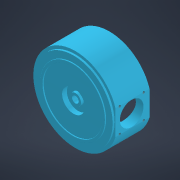
# Autodesk Inventor part: 008
Saved by Autodesk Inventor 2022 (Build 260153000, 153)
## iProperties
Created: 2021-11-17
Part Number: 008
Material: Steel, Carbon
Document SubType Name: Modeling
Designer: vinicius.miguel
Density: 7.85 g/cm^3
Appearance: Turquoise
Mass: 775.835 g
Surface Area: 314.081 cm^2
Volume: 98.8324 cm^3
Author: vinicius.miguel
Autodesk Inventor part; units mm, degrees
ref_plane "XZ Plane" through (0, 0, 0) normal (0, 1, 0) x (-1, 0, 0)
ref_plane "XY Plane" through (0, 0, 0) normal (0, 0, 1) x (1, 0, 0)
sketch "Sketch1" plane through (0, 0, 0) normal (0, 1, 0) x (-1, 0, 0)
  line L0 (0, 0) -> (0, 38)
  line L1 (-3.5, 30) -> (-15, 30)
  line L2 (-15, 30) -> (-15, 35)
  line L3 (-15, 35) -> (-34.45, 35)
  line L4 (-34.45, 35) -> (-34.45, 0)
  line L5 (-34.45, 0) -> (-44.45, 0)
  line L6 (-44.45, 0) -> (-44.45, 38)
  line L7 (-44.45, 38) -> (-34.5, 38)
  line L8 (-34.5, 38) -> (-34.5, 39)
  line L9 (-34.5, 39) -> (-31.5, 39)
  line L10 (-31.5, 39) -> (-31.5, 38)
  line L11 (-31.5, 38) -> (-12, 38)
  line L12 (-12, 33) -> (-3.5, 33)
  line L13 (-12, 38) -> (-12, 33)
  line L14 (-3.5, 33) -> (-3.5, 30)
  line L15 (-3.5, 33) -> (-3.5, 36)
  line L16 (-3.5, 36) -> (-6, 36)
  line L17 (-6, 36) -> (-6, 33)
  dimension "d5" = 69
  dimension "d6" = 3
  dimension "d7" = 1
  dimension "d8" = 88.9
  dimension "d10" = 3
  dimension "d11" = 5
  dimension "d12" = 30
  dimension "d37" = 10
  dimension "d64" = 38
  dimension "d74" = 7
  dimension "d75" = 24
  dimension "d76" = 3
  dimension "d77" = 2.5
  dimension "d78" = 3
  constraints: 36 end point, 16 perpendicular, 4 vertical, 2 horizontal alignment, 2 point on line
  measures "d5" diameter of L8 L0
  measures "d6" distance of L8.end L9.end
  measures "d7" distance of L9.end L10.end
  measures "d8" diameter of L6 L0
  measures "d10" distance between parallel lines of L11 L3
  measures "d11" distance of L1.end L2.end
  measures "d12" diameter of L2 L0
  measures "d37" distance between parallel lines of L6 L4
  measures "d64" distance of L5.end L6.end
  measures "d74" diameter of L14 L0
  measures "d75" diameter of L13 L0
  measures "d76" distance of L12.end L1.start
  measures "d77" distance of L15.end L16.end
  measures "d78" distance of L16.end L17.end
revolve "Revolution1" add sketch "Sketch1" angle 360 about axis through (0, 0, 0) along (0, 0, 1)
ref_plane "Work Plane1" through (44.45, 0, 19) normal (1, 0, 0) x (0, 1, 0)
sketch "Sketch7" plane through (44.45, 0, 19) normal (1, 0, 0) x (0, 1, 0)
  line L0 (34.45, 16) -> (-34.45, 16) projected
  line L1 (34.45, -19) -> (-34.45, -19) projected
  line L2 (34.45, 16) -> (-34.45, 16) projected
  line L3 (0, 16) -> (0, -19) construction
  line L4 (57.5, 28.575) -> (-57.5, 28.575)
  line L5 (-57.5, 28.575) -> (-57.5, -31.575)
  line L6 (-57.5, -31.575) -> (57.5, -31.575)
  line L7 (57.5, -31.575) -> (57.5, 28.575)
  line L8 (57.5, 28.575) -> (-57.5, -31.575) construction
  line L9 (-57.5, 28.575) -> (57.5, -31.575) construction
  point P0 (0, -1.5)
  dimension "d79" = 115
  dimension "d80" = 60.1501
  constraints: 14 end point, 4 midpoint, 2 parallel, 2 perpendicular, 1 horizontal
  measures "d79" distance of L4.start L4.end
  measures "d80" distance of L6.end L4.start
extrude "Extrusion5" cut sketch "Sketch7" against normal blind 4
chamfer "Chamfer1" distance 0.25 angle 45 4 edges at (-44.45, 0, 38) (-34.5, 0, 39) (-31.5, 0, 39) (40.45, 0, 38)
sketch "Sketch8" plane through (40.45, 0, 19) normal (1, 0, 0) x (0, 0, -1)
  circle A0 centre (0.125, 0) radius 12.5
  line L0 (19, 44.45) -> (19, -44.45) projected
  line L1 (-19, -44.2) -> (-19, 44.2) projected
  line L2 (19, -18.4282) -> (-18.75, -18.4282) projected
  point P0 (19, 0)
  point P1 (19, 18.4282)
  point P2 (-19, -18.3739)
  point P3 (-19, 18.3739)
  point P4 (19, 0)
  point P5 (0.125, -18.4282)
  dimension "d44" = 25
  constraints: 2 midpoint, 1 centre point, 1 horizontal alignment, 1 vertical alignment
  measures "d44" diameter of A0
extrude "Extrusion6" cut sketch "Sketch8" against normal blind 20
sketch "Sketch10" plane through (40.45, 0, 19) normal (1, 0, 0) x (0, 0, -1)
  circle A0 centre (0.125, 0) radius 12.5 projected
  line L0 (0.125, 0) -> (19, 0)
  line L1 (19, 18.4282) -> (19, -18.4282) projected
  line L2 (0.125, 0) -> (12.8529, 12.7279)
  point P0 (19, 0)
  dimension "d51" = 18
  dimension "d65" = 45
  constraints: 4 end point, 1 horizontal, 1 midpoint
  measures "d51" distance of L2.end L0.start
  measures "d65" angle of L0 L2
hole "Hole2" at (40.45, 12.7279, 6.1471) direction (-1, 0, 0) diameter 2.459 depth 4.5 tip angle 118 thread size "M3x0.5" class "6H" standard "ISO Metric profile"
pattern_circular "Circular Pattern1" count 4 over 360 about axis through (40.45, 0, 18.875) along (-1, 0, 0) of "Hole2"
sketch "Sketch12" plane through (0, 0, 38) normal (0, 0, 1) x (1, 0, 0)
  circle A0 centre (0, 0) radius 41.45
  circle A1 centre (0, 0) radius 44.45
  point P0 (0, 0)
  dimension "d81" = 82.9
  dimension "d82" = 88.9
  constraints: 2 centre point, 2 coincident
  measures "d81" diameter of A0
  measures "d82" diameter of A1
extrude "Extrusion9" cut sketch "Sketch12" against normal blind 2
body "Solid1"
